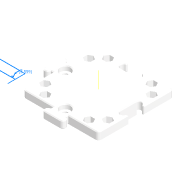
# Autodesk Inventor part: 10_Base_puzzle_cassetteadapter_v3
Saved by Autodesk Inventor 2022 (Build 260153000, 153)
## iProperties
Created: 2017-06-20
Part Number: 10_Base_puzzle_cassetteadapter_v3
Material: Generisch
Document SubType Name: Modeling
Designer: diederichbenedict
Density: 1 g/cm^3
Appearance: Weiß
Mass: 5.4697 g
Surface Area: 48.9743 cm^2
Volume: 5.4697 cm^3
Catalog Web Link: isInjectionmolded
Vendor: openUC2
d_part: 50,000 mm
d_o: 40,000 mm
d_i: 40,000 mm
Author: diederichbenedict
Autodesk Inventor part; units mm, degrees
ref_plane "YZ Plane" through (0, 0, 0) normal (1, 0, 0) x (0, 1, 0)
ref_plane "XZ Plane" through (0, 0, 0) normal (0, 1, 0) x (-1, 0, 0)
ref_plane "XY Plane" through (0, 0, 0) normal (0, 0, 1) x (1, 0, 0)
sketch "Skizze1" plane through (0, 0, 0) normal (0, 0, 1) x (1, 0, 0)
  line L0 (-17, 0) -> (-25, 0)
  line L1 (-25, 0) -> (-25, -23)
  line L2 (-23, -25) -> (0, -25)
  line L3 (0, -25) -> (0, -17)
  line L4 (-17, 0) -> (-17, -15)
  line L5 (-15, -17) -> (0, -17)
  arc A0 (-25, -23) -> (-23, -25) centre (-23, -23) ccw
  circle A1 centre (-20.8, -14.5) radius 2.55 construction
  circle A2 centre (-14.5, -20.8) radius 2.55 construction
  arc A3 (-17, -15) -> (-15, -17) centre (-15, -15) ccw
  circle A4 centre (-14.5, -20.8) radius 2.55 construction
  circle A5 centre (-20.8, -14.5) radius 2.55 construction
  line L6 (-30.4971, 0) -> (5.0828, 0) construction
  line L7 (0, -30.4971) -> (0, 5.0828) construction
  line L8 (-18.25, -13.0278) -> (-18.25, -15.9722)
  line L9 (-18.25, -15.9722) -> (-20.8, -17.4445)
  line L10 (-20.8, -17.4445) -> (-23.35, -15.9722)
  line L11 (-23.35, -15.9722) -> (-23.35, -13.0278)
  line L12 (-23.35, -13.0278) -> (-20.8, -11.5555)
  line L13 (-20.8, -11.5555) -> (-18.25, -13.0278)
  line L14 (-15.9722, -18.25) -> (-13.0278, -18.25)
  line L15 (-13.0278, -18.25) -> (-11.5555, -20.8)
  line L16 (-11.5555, -20.8) -> (-13.0278, -23.35)
  line L17 (-13.0278, -23.35) -> (-15.9722, -23.35)
  line L18 (-15.9722, -23.35) -> (-17.4445, -20.8)
  line L19 (-17.4445, -20.8) -> (-15.9722, -18.25)
  point P0 (-25, -25)
  point P1 (-17, -17)
  dimension "d278" = 25
  dimension "d279" = 25
  dimension "d2" = 8
  dimension "d281" = 8
  dimension "d282" = 2
  dimension "d286" = 5.1
  dimension "d_hole" = 5.1
  dimension "d290" = 20.8
  dimension "d" = 20.8
  dimension "d292" = 2
  dimension "d313" = 6.3
  dimension "d314" = 6.3
  dimension "d331" = 0
  dimension "d332" = 0
  constraints: 36 end point, 6 centre point, 6 tangent, 5 coincident, 4 parallel, 4 point on circle, 4 point on line, 2 collinear, 1 horizontal, 1 perpendicular, 26 other
  measures "d278" distance of L2.end point (-25, -25)
  measures "d279" distance of point (-25, -25) L0.end
  measures "d2" distance between parallel lines of L4 L1
  measures "d281" distance between parallel lines of L2 L5
  measures "d282" radius of A0
  measures "d286" diameter of A1
  measures "d_hole" diameter of A2
  measures "d290" distance from line of L0 A2.centre
  measures "d" distance from line of L3 A1.centre
  measures "d292" radius of A3
  measures "d313" horizontal distance of A1.centre A2.centre
  measures "d314" horizontal distance of A1.centre A2.centre
  measures "d331" radial gap between concentric circles of A2 A4
  measures "d332" radial gap between concentric circles of A1 A5
extrude "Extrusion1" add sketch "Skizze1" along normal blind 5
mirror "Mirror6" about plane through (-17, 0, 0) normal (0, 1, 0) of "Extrusion1"
mirror "Mirror7" about plane through (0, -25, 0) normal (1, 0, 0) of "Extrusion1", "Mirror6"
sketch "Sketch26" plane through (0, 0, 5) normal (0, 0, 1) x (1, 0, 0)
  line L0 (23, 25) -> (-23, 25) projected
  arc A0 (-23, 25) -> (-25, 23) centre (-23, 23) ccw projected
  line L1 (-25, -23) -> (-25, 23) projected
  arc A1 (-25, -23) -> (-23, -25) centre (-23, -23) ccw projected
  line L2 (-23, -25) -> (23, -25) projected
  arc A2 (23, -25) -> (25, -23) centre (23, -23) ccw projected
  line L3 (25, 23) -> (25, -23) projected
  arc A3 (25, 23) -> (23, 25) centre (23, 23) ccw projected
  line L4 (15, 17) -> (-15, 17) projected
  arc A4 (17, 15) -> (15, 17) centre (15, 15) ccw projected
  line L5 (17, 15) -> (17, -15) projected
  arc A5 (15, -17) -> (17, -15) centre (15, -15) ccw projected
  line L6 (-15, -17) -> (15, -17) projected
  arc A6 (-17, -15) -> (-15, -17) centre (-15, -15) ccw projected
  line L7 (-17, -15) -> (-17, 15) projected
  arc A7 (-15, 17) -> (-17, 15) centre (-15, 15) ccw projected
  line L8 (-25, -23) -> (-25, 23) projected
  line L9 (-28.6, -7) -> (-28.6, -7)
  line L10 (-30.6, -5) -> (-30.6, 5)
  line L11 (-28.6, 7) -> (-28.6, 7)
  line L12 (-25, 16.8311) -> (-25, -7)
  line L13 (-26.3639, 5) -> (-25, 5)
  line L14 (-25, -5) -> (-26.3639, -5)
  arc A8 (-30.6, -5) -> (-28.6, -7) centre (-28.6, -5) ccw
  arc A9 (-28.6, -7) -> (-26.6124, -5.2222) centre (-28.6, -5) ccw
  arc A10 (-28.6, 7) -> (-30.6, 5) centre (-28.6, 5) ccw
  arc A11 (-26.6124, 5.2222) -> (-28.6, 7) centre (-28.6, 5) ccw
  arc A12 (-26.3639, -5) -> (-26.6124, -5.2222) centre (-26.3639, -5.25) ccw
  arc A13 (-26.6124, 5.2222) -> (-26.3639, 5) centre (-26.3639, 5.25) ccw
  line L15 (-42.4199, 0) -> (36.7199, 0) projected
  point P0 (0, 0)
  point P1 (-24.0313, 1.861)
  point P2 (-28.6, -7)
  point P3 (-25, -5)
  point P4 (-25, 5)
  point P5 (-28.6, 7)
  dimension "d293" = 5.6
  dimension "d300" = 2
  dimension "d301" = 0.25
  dimension "d365" = 7
  dimension "d367" = 7
  dimension "d385" = 5
  dimension "d386" = 5
  constraints: 12 end point, 12 point on circle, 10 tangent, 6 centre point, 4 equal radius, 3 parallel, 2 coincident, 2 point on line, 1 horizontal, 1 perpendicular, 1 other
  measures "d293" distance between parallel lines of L1 L10
  measures "d300" radius of A8
  measures "d301" radius of A12
  measures "d385" distance of the line from the sketch origin of L14
  measures "d386" distance of the line from the sketch origin of L13
extrude "Extrusion13" add sketch "Sketch26" against normal up to surface (5 mm away) contours L1 L15 L10 A10 A11 A13 L13 | L1 L14 A12 A9 A8 L10 L15
sketch "Sketch28" plane through (0, 0, 5) normal (0, 0, 1) x (1, 0, 0)
  line L0 (-42.0399, 0) -> (37.3035, 0) construction
  line L1 (23, 25) -> (-23, 25) projected
  arc A0 (-23, 25) -> (-25, 23) centre (-23, 23) ccw projected
  line L2 (-25, 5) -> (-25, 23) projected
  arc A1 (-25, -23) -> (-23, -25) centre (-23, -23) ccw projected
  line L3 (-23, -25) -> (23, -25) projected
  arc A2 (23, -25) -> (25, -23) centre (23, -23) ccw projected
  line L4 (25, 23) -> (25, -23) projected
  arc A3 (25, 23) -> (23, 25) centre (23, 23) ccw projected
  line L5 (15, 17) -> (-15, 17) projected
  arc A4 (17, 15) -> (15, 17) centre (15, 15) ccw projected
  line L6 (17, 15) -> (17, -15) projected
  arc A5 (15, -17) -> (17, -15) centre (15, -15) ccw projected
  line L7 (-15, -17) -> (15, -17) projected
  arc A6 (-17, -15) -> (-15, -17) centre (-15, -15) ccw projected
  line L8 (-17, -15) -> (-17, 15) projected
  arc A7 (-15, 17) -> (-17, 15) centre (-15, 15) ccw projected
  line L9 (24.4624, 5.1058) -> (23.9221, 5.1058) construction
  line L10 (19.1833, 5.0625) -> (23.3833, 5.0625) construction
  line L11 (19.1833, 5.0625) -> (23.3833, 5.0625) construction
  line L12 (23.3833, 5.0625) -> (23.4138, 5.032) construction
  line L13 (23.3833, 5.0625) -> (23.7431, 5.0625) construction
  line L14 (25, 5) -> (25, 0.1058)
  line L15 (25, 23) -> (25, -23) projected
  line L16 (24.4624, 5.1058) -> (25, 5.6434) construction
  line L17 (25, 5) -> (25.2369, 5) construction
  line L18 (25, 5.6434) -> (25, 5)
  line L19 (-25, 5) -> (-26.3639, 5) construction
  arc A8 (-26.6124, 5.2222) -> (-26.3639, 5) centre (-26.3639, 5.25) ccw construction
  arc A9 (-26.6124, 5.2222) -> (-30.6, 5) centre (-28.6, 5) ccw construction
  line L20 (-30.6, 5) -> (-30.6, -5) construction
  arc A10 (-30.6, -5) -> (-26.6124, -5.2222) centre (-28.6, -5) ccw construction
  arc A11 (-26.3639, -5) -> (-26.6124, -5.2222) centre (-26.3639, -5.25) ccw construction
  line L21 (-26.3639, -5) -> (-25, -5) construction
  line L22 (-25, -23) -> (-25, -5) projected
  line L23 (24.4624, -5.1058) -> (23.9221, -5.1058) construction
  line L24 (19.1833, -5.0625) -> (23.3833, -5.0625) construction
  line L25 (19.1833, -5.0625) -> (23.3833, -5.0625) construction
  line L26 (23.3833, -5.0625) -> (23.4138, -5.032) construction
  line L27 (23.3833, -5.0625) -> (23.7431, -5.0625) construction
  line L28 (25, -5) -> (25, 0.1058)
  line L29 (24.4624, -5.1058) -> (25, -5.6434) construction
  line L30 (25, -5) -> (25.2369, -5) construction
  line L31 (25, -5.6434) -> (25, -5)
  line L32 (21.3, -6.95) -> (21.3, -6.95) construction
  line L33 (19.3, -4.95) -> (19.3, 5.05) construction
  line L34 (21.3, 7.05) -> (21.3, 7.05) construction
  line L35 (23.5226, 5.1498) -> (25, 5.1497) construction
  line L36 (25, -5.0501) -> (23.5226, -5.05) construction
  arc A12 (19.3, -4.95) -> (21.3, -6.95) centre (21.3, -4.95) ccw construction
  arc A13 (21.3, -6.95) -> (23.2757, -5.2611) centre (21.3, -4.95) ccw construction
  arc A14 (21.3, 7.05) -> (19.3, 5.05) centre (21.3, 5.05) ccw construction
  arc A15 (23.2757, 5.3609) -> (21.3, 7.05) centre (21.3, 5.05) ccw construction
  arc A16 (23.5226, -5.05) -> (23.2757, -5.2611) centre (23.5226, -5.3) ccw construction
  arc A17 (23.2757, 5.3609) -> (23.5226, 5.1498) centre (23.5226, 5.3998) ccw construction
  line L37 (-30.6, 5) -> (-30.6, -5) projected
  line L38 (-25, 5) -> (-26.3639, 5) projected
  line L39 (-25, 5) -> (-26.3639, 5)
  arc A18 (-26.6124, 5.2222) -> (-26.3639, 5) centre (-26.3639, 5.25) ccw projected
  arc A19 (-26.6124, 5.2222) -> (-26.3639, 5) centre (-26.3639, 5.25) ccw
  arc A20 (-26.6124, 5.2222) -> (-30.6, 5) centre (-28.6, 5) ccw
  line L40 (-30.6, 5) -> (-30.6, 0)
  line L41 (25, 5.1497) -> (23.4675, 5.1498)
  arc A21 (23.4675, 5.1498) -> (19.55, 5.05) centre (21.51, 5.05) ccw
  line L42 (19.55, 5.05) -> (19.55, 0)
  line L43 (24.4624, -5.1058) -> (23.9221, -5.1058) construction
  line L44 (19.1833, -5.0625) -> (23.3833, -5.0625) construction
  line L45 (19.1833, -5.0625) -> (23.3833, -5.0625) construction
  line L46 (23.3833, -5.0625) -> (23.4138, -5.032) construction
  line L47 (23.3833, -5.0625) -> (23.7431, -5.0625) construction
  line L48 (25, -5) -> (25, -0.1058)
  line L49 (24.4624, -5.1058) -> (25, -5.6434) construction
  line L50 (25, -5) -> (25.2369, -5) construction
  line L51 (25, -5.6434) -> (25, -5)
  arc A22 (23.5226, -5.1498) -> (23.2757, -5.3609) centre (23.5226, -5.3998) ccw construction
  arc A23 (21.3, -7.05) -> (23.2757, -5.3609) centre (21.3, -5.05) ccw construction
  line L52 (23.5226, -5.1498) -> (25, -5.1497) construction
  arc A24 (19.3, -5.05) -> (21.3, -7.05) centre (21.3, -5.05) ccw construction
  line L53 (25, -5.1497) -> (23.4675, -5.1498)
  arc A25 (19.55, -5.05) -> (23.4675, -5.1498) centre (21.51, -5.05) ccw
  arc A26 (23.4675, -5.1498) -> (23.4675, -5.1498) centre (23.3175, -5.15) ccw
  line L54 (19.55, -5.05) -> (19.55, 0)
  line L55 (19.55, 0) -> (25, 0)
  point P0 (23.3495, 5.1058)
  point P1 (23.3495, -5.1058)
  point P2 (25, -7)
  point P3 (25.9687, 1.861)
  point P4 (23.3495, -5.1058)
  point P5 (25.9687, -1.861)
  point P6 (23.4675, -5.1498)
  dimension "d22" = 0
  dimension "d23" = 0
  dimension "d369" = 4.2
  dimension "d370" = 0
  dimension "d380" = 45
  dimension "d387" = 2
  dimension "d388" = 0.25
  dimension "d391" = 0.1
  dimension "d392" = 5.05
  dimension "d393" = 5.05
  dimension "d394" = 1.96
  dimension "d396" = 5.45
  dimension "d397" = 7.05
  constraints: 80 end point, 30 symmetric about line, 28 point on circle, 14 centre point, 14 tangent, 8 point on line, 5 horizontal, 4 collinear, 4 equal radius, 3 coincident, 2 parallel, 2 perpendicular, 1 midpoint, 4 other
  measures "d369" distance of L10.start L10.end
  measures "d370" distance between parallel lines of L10 L11
  measures "d380" angle of L17 L16
  measures "d387" radius of A12
  measures "d388" radius of A16
  measures "d391" distance from line of L35 A15.centre
  measures "d392" distance from line of L0 A15.centre
  measures "d393" distance from line of L0 A21.centre
  measures "d394" radius of A21
  measures "d396" distance between parallel lines of L4 L42
  measures "d397" distance from line of L0 L34.end
extrude "Extrusion14" cut sketch "Sketch28" against normal blind 10 contours L4 L55 L42 A21 L41 | A26 | L4 L53 A25 L54 L55
pattern_circular "Circular Pattern6" count 2 over 90 about axis through (0, 0, 5) along (0, 0, 1) of "Extrusion14", "Extrusion13"
sketch "Sketch29" plane through (0, 0, 5) normal (0, 0, 1) x (1, 0, 0)
  arc A0 (-23, 25) -> (-25, 23) centre (-23, 23) ccw projected
  line L0 (-25, 5) -> (-25, 23) projected
  arc A1 (-25, -23) -> (-23, -25) centre (-23, -23) ccw projected
  line L1 (-23, -25) -> (-5, -25) projected
  arc A2 (23, -25) -> (25, -23) centre (23, -23) ccw projected
  arc A3 (25, 23) -> (23, 25) centre (23, 23) ccw projected
  line L2 (15, 17) -> (-15, 17) projected
  arc A4 (17, 15) -> (15, 17) centre (15, 15) ccw projected
  line L3 (17, 15) -> (17, -15) projected
  arc A5 (15, -17) -> (17, -15) centre (15, -15) ccw projected
  line L4 (-15, -17) -> (15, -17) projected
  arc A6 (-17, -15) -> (-15, -17) centre (-15, -15) ccw projected
  line L5 (-17, -15) -> (-17, 15) projected
  arc A7 (-15, 17) -> (-17, 15) centre (-15, 15) ccw projected
  circle A8 centre (-22, 0) radius 3.89
  circle A9 centre (0, -22) radius 2.9259
  line L6 (-41.929, 0) -> (36.6381, 0) construction
  line L7 (0, -41.929) -> (0, 36.6381) construction
  line L8 (25, -5.1497) -> (25, -23) projected
  line L9 (-5.1497, 25) -> (-23, 25) projected
  line L10 (-25, 5) -> (-26.3639, 5) projected
  arc A10 (-26.6124, 5.2222) -> (-26.3639, 5) centre (-26.3639, 5.25) ccw projected
  arc A11 (-26.6124, 5.2222) -> (-30.6, 5) centre (-28.6, 5) ccw projected
  line L11 (-30.6, 5) -> (-30.6, -5) projected
  arc A12 (-30.6, -5) -> (-26.6124, -5.2222) centre (-28.6, -5) ccw projected
  arc A13 (-26.3639, -5) -> (-26.6124, -5.2222) centre (-26.3639, -5.25) ccw projected
  line L12 (-26.3639, -5) -> (-25, -5) projected
  line L13 (-25, -23) -> (-25, -5) projected
  line L14 (-5, -25) -> (-5, -26.3639) projected
  arc A14 (-5.2222, -26.6124) -> (-5, -26.3639) centre (-5.25, -26.3639) ccw projected
  arc A15 (-5.2222, -26.6124) -> (-5, -30.6) centre (-5, -28.6) ccw projected
  line L15 (-5, -30.6) -> (5, -30.6) projected
  arc A16 (5, -30.6) -> (5.2222, -26.6124) centre (5, -28.6) ccw projected
  arc A17 (5, -26.3639) -> (5.2222, -26.6124) centre (5.25, -26.3639) ccw projected
  line L16 (5, -26.3639) -> (5, -25) projected
  line L17 (5, -25) -> (23, -25) projected
  line L18 (-5.1498, 23.4675) -> (-5.1497, 25) projected
  line L19 (25, -5.1497) -> (23.4675, -5.1498) projected
  arc A18 (19.55, -5.05) -> (23.4675, -5.1498) centre (21.51, -5.05) ccw projected
  line L20 (19.55, -5.05) -> (19.55, 5.05) projected
  arc A19 (23.4675, 5.1498) -> (19.55, 5.05) centre (21.51, 5.05) ccw projected
  line L21 (23.4675, 5.1498) -> (25, 5.1497) projected
  line L22 (25, 23) -> (25, 5.1497) projected
  line L23 (23, 25) -> (5.1497, 25) projected
  line L24 (5.1497, 25) -> (5.1498, 23.4675) projected
  arc A20 (5.05, 19.55) -> (5.1498, 23.4675) centre (5.05, 21.51) ccw projected
  line L25 (5.05, 19.55) -> (-5.05, 19.55) projected
  arc A21 (-5.1498, 23.4675) -> (-5.05, 19.55) centre (-5.05, 21.51) ccw projected
  point P0 (0, 0)
  dimension "d319" = 7.78
  dimension "d320" = 5
  dimension "d322" = 5
  constraints: 2 centre point, 2 point on line, 1 coincident
  measures "d319" diameter of A8
  measures "d320" distance from line of A8.centre L5
  measures "d322" distance from line of L4 A9.centre
hole "Hole7" at (-22, 0, 5) at (0, -22, 5) direction (0, 0, -1) diameter 3.2 end through all counterbore diameter 7 counterbore depth 3
chamfer "Fase4" distance 0.5 angle 45 67 edges at (-28.7113, -6.9969, 5) (-26.5306, -5.0637, 5) (-25.682, -5, 5) (-30.6, 0, 5) (-28.7113, 6.9969, 5) (-26.5306, 5.0637, 5) (-25.682, 5, 5) (-25, -14, 5) (-24.4142, -24.4142, 5) (-14, -25, 5) (0, -30.6, 5) (6.9969, -28.7113, 5) (5.0637, -26.5306, 5) (5, -25.682, 5) (-6.9969, -28.7113, 5) (-5.0637, -26.5306, 5) (-5, -25.682, 5) (0, -18.5, 5) (-22, 3.5, 5) (-25, -14, 0) (-24.4142, -24.4142, 0) (-14, -25, 0) (-17, 0, 0) (-16.4142, 16.4142, 0) (0, 17, 0) (16.4142, 16.4142, 0) (17, 0, 0) (16.4142, -16.4142, 0) (0, -17, 0) (-16.4142, -16.4142, 0) (0, -17, 5) (16.4142, -16.4142, 5) (17, 0, 5) (16.4142, 16.4142, 5) (0, 17, 5) (-16.4142, 16.4142, 5) (-17, 0, 5) (-16.4142, -16.4142, 5) (-26.5306, -5.0637, 0) (-28.7113, -6.9969, 0) (-30.6, 0, 0) (-28.7113, 6.9969, 0) (-26.5306, 5.0637, 0) (-25.682, 5, 0) (-25.682, -5, 0) (6.9969, -28.7113, 0) (0, -30.6, 0) (-6.9969, -28.7113, 0) (-5.0637, -26.5306, 0) (-5, -25.682, 0) (5.0637, -26.5306, 0) (5, -25.682, 0) (-14.0748, 25, 0) (-24.4142, 24.4142, 0) (-25, 14, 0) (14.0748, 25, 0) (24.4142, 24.4142, 0) (25, 14.0748, 0) (25, 14.0748, 5) (24.4142, 24.4142, 5) (14.0748, 25, 5) (25, -14.0748, 5) (24.4142, -24.4142, 5) (14, -25, 5) (-14.0748, 25, 5) (-24.4142, 24.4142, 5) (-25, 14, 5)
fillet "Rundung5" radius 0.75 22 edges at (0, 19.55, 5) (-7.0094, 21.4601, 5) (-5.1498, 23.9837, 5) (5.1498, 23.9837, 5) (7.0094, 21.4601, 5) (21.4601, 7.0094, 5) (23.9837, 5.1498, 5) (21.4601, -7.0094, 5) (23.9837, -5.1498, 5) (19.55, 0, 5) (7.0094, 21.4601, 0) (5.1498, 23.9837, 0) (-7.0094, 21.4601, 0) (-5.1498, 23.9837, 0) (0, 19.55, 0) (25, 5.1497, 2.5) (-5.1497, 25, 2.5) (5.1497, 25, 2.5) (-5.1498, 23.4675, 2.5) (5.1498, 23.4675, 2.5) (23.4675, 5.1498, 2.5) (23.4675, -5.1498, 2.5)
sketch "Skizze33" plane through (0, 0, 5) normal (0, 0, 1) x (1, 0, 0)
  line L0 (12.3234, 28.65) -> (10.7701, 12.4434)
  line L1 (10.7701, 12.4434) -> (-8.1827, 12.4434)
  line L2 (-8.1827, 12.4434) -> (-14.4699, 29.3004)
  line L3 (-14.4699, 29.3004) -> (12.3234, 28.65)
  point P0 (0, 0)
  constraints: 8 end point
extrude "Extrusion18" [suppressed]
sketch "Skizze34" plane through (0, 0, 0) normal (0, 0, -1) x (-1, 0, 0)
  line L0 (20.8, -17.4445) -> (18.25, -15.9722) projected
  line L1 (18.25, -15.9722) -> (18.25, -13.0278) projected
  line L2 (18.25, -13.0278) -> (20.8, -11.5555) projected
  line L3 (20.8, -11.5555) -> (23.35, -13.0278) projected
  line L4 (23.35, -13.0278) -> (23.35, -15.9722) projected
  line L5 (23.35, -15.9722) -> (20.8, -17.4445) projected
  line L6 (11.5555, -20.8) -> (13.0278, -18.25) projected
  line L7 (13.0278, -18.25) -> (15.9722, -18.25) projected
  line L8 (15.9722, -18.25) -> (17.4445, -20.8) projected
  line L9 (17.4445, -20.8) -> (15.9722, -23.35) projected
  line L10 (15.9722, -23.35) -> (13.0278, -23.35) projected
  line L11 (13.0278, -23.35) -> (11.5555, -20.8) projected
  line L12 (11.5555, 20.8) -> (13.0278, 18.25) projected
  line L13 (13.0278, 23.35) -> (11.5555, 20.8) projected
  line L14 (15.9722, 23.35) -> (13.0278, 23.35) projected
  line L15 (17.4445, 20.8) -> (15.9722, 23.35) projected
  line L16 (15.9722, 18.25) -> (17.4445, 20.8) projected
  line L17 (13.0278, 18.25) -> (15.9722, 18.25) projected
  line L18 (20.8, 17.4445) -> (18.25, 15.9722) projected
  line L19 (23.35, 15.9722) -> (20.8, 17.4445) projected
  line L20 (23.35, 13.0278) -> (23.35, 15.9722) projected
  line L21 (20.8, 11.5555) -> (23.35, 13.0278) projected
  line L22 (18.25, 13.0278) -> (20.8, 11.5555) projected
  line L23 (18.25, 15.9722) -> (18.25, 13.0278) projected
  line L24 (-11.5555, -20.8) -> (-13.0278, -18.25) projected
  line L25 (-13.0278, -23.35) -> (-11.5555, -20.8) projected
  line L26 (-15.9722, -23.35) -> (-13.0278, -23.35) projected
  line L27 (-17.4445, -20.8) -> (-15.9722, -23.35) projected
  line L28 (-15.9722, -18.25) -> (-17.4445, -20.8) projected
  line L29 (-13.0278, -18.25) -> (-15.9722, -18.25) projected
  line L30 (-20.8, -17.4445) -> (-18.25, -15.9722) projected
  line L31 (-23.35, -15.9722) -> (-20.8, -17.4445) projected
  line L32 (-23.35, -13.0278) -> (-23.35, -15.9722) projected
  line L33 (-20.8, -11.5555) -> (-23.35, -13.0278) projected
  line L34 (-18.25, -13.0278) -> (-20.8, -11.5555) projected
  line L35 (-18.25, -15.9722) -> (-18.25, -13.0278) projected
  line L36 (-11.5555, 20.8) -> (-13.0278, 18.25) projected
  line L37 (-13.0278, 18.25) -> (-15.9722, 18.25) projected
  line L38 (-15.9722, 18.25) -> (-17.4445, 20.8) projected
  line L39 (-17.4445, 20.8) -> (-15.9722, 23.35) projected
  line L40 (-15.9722, 23.35) -> (-13.0278, 23.35) projected
  line L41 (-13.0278, 23.35) -> (-11.5555, 20.8) projected
  line L42 (-20.8, 17.4445) -> (-18.25, 15.9722) projected
  line L43 (-18.25, 15.9722) -> (-18.25, 13.0278) projected
  line L44 (-18.25, 13.0278) -> (-20.8, 11.5555) projected
  line L45 (-20.8, 11.5555) -> (-23.35, 13.0278) projected
  line L46 (-23.35, 13.0278) -> (-23.35, 15.9722) projected
  line L47 (-23.35, 15.9722) -> (-20.8, 17.4445) projected
  circle A0 centre (0, -22) radius 1.6 projected
  circle A1 centre (22, 0) radius 1.6 projected
  line L48 (17.5, -15) -> (17.5, 15) projected
  arc A2 (15, -17.5) -> (17.5, -15) centre (15, -15) ccw projected
  line L49 (-15, -17.5) -> (15, -17.5) projected
  arc A3 (-17.5, -15) -> (-15, -17.5) centre (-15, -15) ccw projected
  line L50 (-17.5, 15) -> (-17.5, -15) projected
  arc A4 (-15, 17.5) -> (-17.5, 15) centre (-15, 15) ccw projected
  line L51 (15, 17.5) -> (-15, 17.5) projected
  arc A5 (17.5, 15) -> (15, 17.5) centre (15, 15) ccw projected
  arc A6 (-24.5, 5.1926) -> (-24.2499, 5.1498) centre (-24.25, 5.8998) ccw projected
  line L52 (-24.2499, 5.1498) -> (-24.0833, 5.1498) projected
  arc A7 (-24.0833, 5.1498) -> (-23.3711, 5.6646) centre (-24.0833, 5.8998) ccw projected
  arc A8 (-19.55, 5.05) -> (-23.3711, 5.6646) centre (-21.51, 5.05) ccw projected
  line L53 (-19.55, 5.05) -> (-19.55, -5.05) projected
  arc A9 (-23.3711, -5.6646) -> (-19.55, -5.05) centre (-21.51, -5.05) ccw projected
  arc A10 (-23.3711, -5.6646) -> (-24.0833, -5.1498) centre (-24.0833, -5.8998) ccw projected
  line L54 (-24.0833, -5.1498) -> (-25, -5.1497) projected
  line L55 (-25, -5.1497) -> (-25, -23) projected
  arc A11 (-25, -23) -> (-23, -25) centre (-23, -23) ccw projected
  line L56 (-4.5, -25) -> (-23, -25) projected
  line L57 (-4.5, -26.3639) -> (-4.5, -25) projected
  arc A12 (-5.1667, -27.1093) -> (-4.5, -26.3639) centre (-5.25, -26.3639) ccw projected
  arc A13 (-5.1667, -27.1093) -> (-5, -30.1) centre (-5, -28.6) ccw projected
  line L58 (5, -30.1) -> (-5, -30.1) projected
  arc A14 (5, -30.1) -> (5.1667, -27.1093) centre (5, -28.6) ccw projected
  arc A15 (4.5, -26.3639) -> (5.1667, -27.1093) centre (5.25, -26.3639) ccw projected
  line L59 (4.5, -24.5) -> (4.5, -26.3639) projected
  line L60 (23, -24.5) -> (4.5, -24.5) projected
  arc A16 (23, -24.5) -> (24.5, -23) centre (23, -23) ccw projected
  line L61 (24.5, -4.5) -> (24.5, -23) projected
  line L62 (26.3639, -4.5) -> (24.5, -4.5) projected
  arc A17 (27.1093, -5.1667) -> (26.3639, -4.5) centre (26.3639, -5.25) ccw projected
  arc A18 (27.1093, -5.1667) -> (30.1, -5) centre (28.6, -5) ccw projected
  line L63 (30.1, 5) -> (30.1, -5) projected
  arc A19 (30.1, 5) -> (27.1093, 5.1667) centre (28.6, 5) ccw projected
  arc A20 (26.3639, 4.5) -> (27.1093, 5.1667) centre (26.3639, 5.25) ccw projected
  line L64 (24.5, 4.5) -> (26.3639, 4.5) projected
  line L65 (24.5, 23) -> (24.5, 4.5) projected
  arc A21 (24.5, 23) -> (23, 24.5) centre (23, 23) ccw projected
  line L66 (5.8997, 24.5) -> (23, 24.5) projected
  line L67 (5.8998, 24.0833) -> (5.8997, 24.5) projected
  arc A22 (5.05, 18.8) -> (5.8998, 24.0833) centre (5.05, 21.51) ccw projected
  line L68 (-5.05, 18.8) -> (5.05, 18.8) projected
  arc A23 (-5.8998, 24.0833) -> (-5.05, 18.8) centre (-5.05, 21.51) ccw projected
  line L69 (-5.8997, 24.5) -> (-5.8998, 24.0833) projected
  line L70 (-23, 24.5) -> (-5.8997, 24.5) projected
  arc A24 (-23, 24.5) -> (-24.5, 23) centre (-23, 23) ccw projected
  line L71 (-24.5, 5.1926) -> (-24.5, 23) projected
  point P0 (0, 0)
extrude "Extrusion19" add sketch "Skizze34" against normal up to surface (5 mm away) contours A2 L49 A3 L50 A4 L51 A5 L48
ref_plane "Arbeitsebene14" through (4.6366, 4.35, -1.7321) normal (0, 1, 0) x (1, 0, 0)
sketch "Skizze35" plane through (4.6366, 4.35, -1.7321) normal (0, 1, 0) x (1, 0, 0)
  arc A0 (8.8108, -1.7321) -> (9.2438, -0.9821) centre (8.8108, -1.2321) ccw projected
  line L0 (-8.8108, -1.7321) -> (8.8108, -1.7321) projected
  arc A1 (-9.2438, -0.9821) -> (-8.8108, -1.7321) centre (-8.8108, -1.2321) ccw projected
  line L1 (-7.7438, 1.616) -> (-9.2438, -0.9821) projected
  arc A2 (-7.7438, 1.616) -> (-7.6768, 1.866) centre (-8.1768, 1.866) ccw projected
  line L2 (-7.6768, 4.7321) -> (-7.6768, 1.866) projected
  line L3 (7.6768, 4.7321) -> (-7.6768, 4.7321) projected
  line L4 (7.6768, 1.866) -> (7.6768, 4.7321) projected
  arc A3 (7.6768, 1.866) -> (7.7438, 1.616) centre (8.1768, 1.866) ccw projected
  line L5 (9.2438, -0.9821) -> (7.7438, 1.616) projected
  line L6 (-27.6366, -1.7321) -> (-9.1366, -1.7321) projected
  line L7 (8.3911, -1.7321) -> (11.3356, -1.7321) projected
  line L8 (11.3356, -1.7321) -> (11.3356, -6.7321) projected
  arc A4 (-7.8304, 1.666) -> (-7.7768, 1.866) centre (-8.1768, 1.866) ccw
  line L9 (-7.8304, 1.666) -> (-9.3304, -0.9321)
  arc A5 (-9.3304, -0.9321) -> (-8.8108, -1.8321) centre (-8.8108, -1.2321) ccw
  line L10 (-8.8108, -1.8321) -> (8.8108, -1.8321)
  arc A6 (8.8108, -1.8321) -> (9.3304, -0.9321) centre (8.8108, -1.2321) ccw
  line L11 (9.3304, -0.9321) -> (7.8304, 1.666)
  arc A7 (7.7768, 1.866) -> (7.8304, 1.666) centre (8.1768, 1.866) ccw
  line L12 (7.7768, 1.866) -> (7.7768, 4.8321)
  line L13 (7.7768, 4.8321) -> (-7.7768, 4.8321)
  line L14 (-7.7768, 4.8321) -> (-7.7768, 1.866)
  line L15 (7.7768, 4.7321) -> (11.3356, 4.7321)
  line L16 (11.3356, 4.7321) -> (11.3356, -1.7321)
  line L17 (-7.7768, 4.7321) -> (-11.3356, 4.7321)
  line L18 (-11.3356, 4.7321) -> (-11.3356, -1.7321)
  line L19 (14.9134, -5.9821) -> (14.9134, -1.7321) projected
  line L20 (11.3356, 4.7321) -> (14.9134, -1.7321)
  line L21 (11.3356, -1.7321) -> (12.8078, -1.7321) projected
  line L22 (11.3356, -1.7321) -> (14.9134, -1.7321)
  line L23 (-11.3356, 4.7321) -> (-14.6402, -1.7321)
  line L24 (-11.3356, -1.7321) -> (-14.6402, -1.7321)
  point P0 (-4.6366, -1.7321)
  point P1 (9.1425, -1.7321)
  point P2 (-9.1425, -1.7321)
  dimension "d403" = 0.1
  dimension "d404" = 3.5588
  dimension "d405" = 3.5588
  constraints: 28 end point, 8 point on circle, 6 point on line, 4 centre point, 2 collinear, 2 perpendicular, 1 horizontal, 9 other
  measures "d403" distance between parallel lines of L2 L14
  measures "d404" distance between parallel lines of L16 L12
  measures "d405" distance between parallel lines of L18 L14
extrude "Extrusion20" add sketch "Skizze35" along normal blind 5 and the other way blind 15 contours L23 L18 L6 | L18 L17 L14 A4 L9 A5 L6 | A6 L11 A7 L12 L15 L16 L7 | L16 L20 L22 L21
equation "\"d22\" = 0"
equation "\"d23\" = 0"
equation "\"d_i\" = 40"
equation "\"d_o\" = 40"
equation "\"d_part\" = 50"
equation "\"d6\" = 0"
equation "\"d7\" = 0"
equation "\"d8\" = 0"
equation "\"d9\" = 0"
equation "\"d13\" = 0"
equation "\"d14\" = 0"
equation "\"d20\" = 0"
equation "\"d21\" = 0"
equation "\"d24\" = 0"
equation "\"d25\" = 3"
equation "\"d26\" = 0"
equation "\"d27\" = 0"
equation "\"d28\" = 0"
equation "\"d29\" = 0"
equation "\"d30\" = 0"
equation "\"d31\" = 0"
equation "\"d32\" = 0"
equation "\"d33\" = 0"
equation "\"d34\" = 0"
equation "\"d46\" = 0"
equation "\"d47\" = 0"
equation "\"d48\" = 0"
equation "\"d50\" = 0"
equation "\"d51\" = 0"
equation "\"d52\" = 0"
equation "\"d53\" = 0"
equation "\"d54\" = 0"
equation "\"d55\" = 0"
equation "\"d56\" = 0"
equation "\"d57\" = 0"
equation "\"d58\" = 0"
equation "\"d59\" = 0"
equation "\"magnet_offset\" = 0"
equation "\"screw_offset\" = 0"
equation "\"mal_puzzle_offset\" = 0"
equation "\"fem_puzzle_offset\" = 0"
